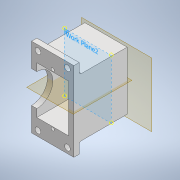
# Autodesk Inventor part: peristaltic pump bracket
Saved by Autodesk Inventor 2022 (Build 260153000, 153)
## iProperties
Created: 2022-01-06
Part Number: peristaltic pump bracket
Material: Generic
Document SubType Name: Modeling
Designer: efred
Density: 1 g/cm^3
Appearance: Default
Author: efred
Autodesk Inventor part; units mm, degrees
ref_plane "YZ Plane" through (0, 0, 0) normal (1, 0, 0) x (0, 1, 0)
ref_plane "XZ Plane" through (0, 0, 0) normal (0, 1, 0) x (-1, 0, 0)
ref_plane "XY Plane" through (0, 0, 0) normal (0, 0, 1) x (1, 0, 0)
ref_plane "Work Plane1" through (0, 0, 0) normal (0, 0, 1) x (1, 0, 0)
sketch "Sketch1" plane through (0, 0, 0) normal (0, 0, 1) x (1, 0, 0)
  circle A0 centre (0, 24.15) radius 1.6 construction
  circle A1 centre (0, -24.15) radius 1.6 construction
  line L0 (-19.85, -7.6776) -> (-19.85, 7.6776) construction
  arc A2 (-19.85, -7.6776) -> (-19.2715, -9.0845) centre (-17.85, -7.6776) ccw construction
  line L1 (-2.2034, -26.3306) -> (-19.2715, -9.0845) construction
  arc A3 (-2.2034, -26.3306) -> (2.2034, -26.3306) centre (0, -24.15) ccw construction
  line L2 (19.2715, -9.0845) -> (2.2034, -26.3306) construction
  arc A4 (19.2715, -9.0845) -> (19.85, -7.6776) centre (17.85, -7.6776) ccw construction
  line L3 (19.85, 7.6776) -> (19.85, -7.6776) construction
  arc A5 (19.85, 7.6776) -> (19.2715, 9.0845) centre (17.85, 7.6776) ccw construction
  line L4 (2.2034, 26.3306) -> (19.2715, 9.0845) construction
  arc A6 (2.2034, 26.3306) -> (-2.2034, 26.3306) centre (0, 24.15) ccw construction
  line L5 (-19.2715, 9.0845) -> (-2.2034, 26.3306) construction
  arc A7 (-19.2715, 9.0845) -> (-19.85, 7.6776) centre (-17.85, 7.6776) ccw construction
  circle A8 centre (0, 0) radius 13.8 construction
  circle A9 centre (0, 0) radius 14.3 construction
  line L6 (-19.85, -27.25) -> (19.85, -27.25)
  line L7 (19.85, -27.25) -> (19.85, 27.25)
  line L8 (19.85, 27.25) -> (-19.85, 27.25)
  line L9 (-19.85, 27.25) -> (-19.85, -27.25)
  circle A10 centre (0, -24.15) radius 1.5
  circle A11 centre (0, 24.15) radius 1.5
  line L10 (14.85, 22.25) -> (14.85, -22.25)
  line L11 (14.85, -22.25) -> (-14.85, -22.25)
  line L12 (-14.85, -22.25) -> (-14.85, 22.25)
  line L13 (-14.85, 22.25) -> (14.85, 22.25)
  dimension "d0" = 0.5
  dimension "d2" = 3
  dimension "d3" = 3
  dimension "d4" = 5
  constraints: 16 end point, 4 parallel, 3 centre point, 2 coincident, 2 collinear, 2 perpendicular, 2 tangent, 1 horizontal, 3 other
  measures "d0" radial gap between concentric circles of A8 A9
  measures "d2" diameter of A10
  measures "d3" diameter of A11
  measures "d4" distance between parallel lines of L7 L10
extrude "Extrusion1" add sketch "Sketch1" along normal blind 50
sketch "Sketch2" plane through (-19.85, -27.25, 0) normal (-1, 0, 0) x (0, 0, 1)
  line L0 (50, 54.5) -> (50, 0) projected
  line L1 (50, 0) -> (50, 54.5) projected
  circle A0 centre (50, 27.25) radius 15
  point P0 (0, 27.25)
  point P1 (50, 12.25)
  point P2 (50, 42.25)
  dimension "d7" = 30
  constraints: 1 centre point, 1 midpoint
  measures "d7" diameter of A0
extrude "Extrusion2" cut sketch "Sketch2" against normal up to surface (34.7 mm away) contours L0 A0 picked at (45.0365, 27.8527)
sketch "Sketch3" plane through (0, 0, 50) normal (0, 0, 1) x (1, 0, 0)
  line L0 (19.85, 27.25) -> (-19.85, 27.25) projected
  line L1 (-19.85, 27.25) -> (19.85, 27.25)
  line L2 (19.85, 27.25) -> (19.85, 37.25)
  line L3 (19.85, 37.25) -> (-19.85, 37.25)
  line L4 (-19.85, 37.25) -> (-19.85, 27.25)
  line L5 (19.85, -27.25) -> (19.85, 27.25) projected
  circle A0 centre (-13.85, 32.25) radius 2.65
  circle A1 centre (13.85, 32.25) radius 2.65
  line L6 (0, 37.25) -> (0, 27.25) construction
  point P0 (0, 0)
  point P1 (-19.85, 32.25)
  dimension "d10" = 5.3
  dimension "d12" = 6
  dimension "d13" = 10
  constraints: 10 end point, 3 midpoint, 2 centre point, 2 parallel, 1 collinear, 1 horizontal, 1 horizontal alignment, 1 perpendicular, 1 other
  measures "d10" diameter of A0
  measures "d12" distance from line of L4 A0.centre
  measures "d13" distance between parallel lines of L0 L3
extrude "Extrusion3" add sketch "Sketch3" against normal blind 5
fillet "Fillet1" radius 2 1 edges at (0, 27.25, 45)
ref_plane "Work Plane2" through (-19.85, 0, 0) normal (0, 1, 0) x (1, 0, 0)
mirror "Mirror1" about plane through (-19.85, 0, 0) normal (0, 1, 0) of "Extrusion3", "Fillet1"
body "Solid1"
